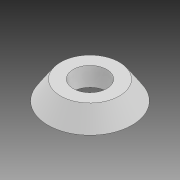
# Autodesk Inventor part: PulleySpacer
Saved by Autodesk Inventor 2020 (Build 240168000, 168)
## iProperties
Created: 2020-08-23
Part Number: PulleySpacer
Material: Generic
Document SubType Name: Modeling
Designer: DDeGo
Density: 1 g/cm^3
Appearance: Default
Author: DDeGo
Autodesk Inventor part; units mm, degrees
ref_plane "YZ Plane" through (0, 0, 0) normal (1, 0, 0) x (0, 1, 0)
ref_plane "XZ Plane" through (0, 0, 0) normal (0, 1, 0) x (-1, 0, 0)
ref_plane "XY Plane" through (0, 0, 0) normal (0, 0, 1) x (1, 0, 0)
sketch "Sketch1" plane through (0, 0, 0) normal (0, 0, 1) x (1, 0, 0)
  line L0 (0, 0) -> (0, 3) construction
  line L1 (0, 3) -> (2.65, 3) construction
  line L2 (2.65, 3) -> (2.65, 0)
  line L3 (2.65, 0) -> (0, 0) construction
  line L4 (2.65, 0) -> (6.65, 0)
  line L5 (6.65, 0) -> (4.65, 3)
  line L6 (4.65, 3) -> (2.65, 3)
  dimension "d0" = 2.65
  dimension "d1" = 3
  dimension "d2" = 2
  dimension "d3" = 4
  constraints: 14 end point, 3 perpendicular, 2 point on line, 1 parallel, 1 vertical
  measures "d0" distance between parallel lines of L0 L2
  measures "d1" distance between parallel lines of L4 L6
  measures "d2" distance of L5.end L1.end
  measures "d3" distance of L2.end L4.end
revolve "Revolution1" add sketch "Sketch1" angle 360 about axis through (0, 0, 0) along (0, 1, 0)
body "Solid1"
